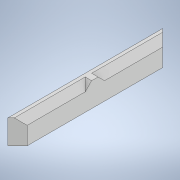
# Autodesk Inventor part: edge-join-no-hole
Saved by Autodesk Inventor 2021 (Build 250183000, 183)
## iProperties
Created: 2020-12-10
Part Number: edge-join-no-hole
Material: Generic
Document SubType Name: Modeling
Designer: Luke Kamols
Density: 1 g/cm^3
Appearance: Default
Author: Luke Kamols
Autodesk Inventor part; units mm, degrees
ref_plane "YZ Plane" through (0, 0, 0) normal (1, 0, 0) x (0, 1, 0)
ref_plane "XZ Plane" through (0, 0, 0) normal (0, 1, 0) x (-1, 0, 0)
ref_plane "XY Plane" through (0, 0, 0) normal (0, 0, 1) x (1, 0, 0)
sketch "Sketch1" plane through (0, 0, 0) normal (0, 0, 1) x (1, 0, 0)
  line L0 (0, 0) -> (6, 0)
  line L1 (6, 0) -> (6, 11)
  line L2 (0, 0) -> (0, 15)
  line L3 (0, 15) -> (2, 15)
  line L4 (2, 15) -> (6, 11)
  dimension "d0" = 6
  dimension "d1" = 11
  dimension "d2" = 15
  dimension "d3" = 2
  constraints: 10 end point, 2 perpendicular, 1 horizontal, 1 vertical
  measures "d0" distance of L0.start L0.end
  measures "d1" distance of L0.end L1.end
  measures "d2" distance of L0.start L2.end
  measures "d3" distance of L2.end L3.end
extrude "Extrusion1" add sketch "Sketch1" along normal blind 96
sketch "Sketch2" plane through (0, 0, 0) normal (0, -1, 0) x (1, 0, 0)
  line L0 (0, 0) -> (0, 96) projected
  line L1 (5.9866, 0) -> (0, 0)
  line L2 (0, 96) -> (6, 96) projected
  line L3 (0, 96) -> (6, 96)
  line L4 (6, 96) -> (6, 90)
  line L5 (6, 90) -> (0, 96)
  line L6 (0, 0) -> (6, 0) projected
  line L7 (6, 0) -> (0, 0)
  line L8 (6, 0) -> (6, 6)
  line L9 (6, 0) -> (6, 96) projected
  line L10 (6, 6) -> (0, 0)
  dimension "d7" = 6
  dimension "d8" = 6
  constraints: 14 end point, 2 horizontal, 1 collinear, 1 point on line
  measures "d7" distance of L2.end L4.end
  measures "d8" distance of L6.end L8.end
extrude "Extrusion2" cut sketch "Sketch2" against normal blind 42.1125 contours L10 L8 L6 L1 | L2 L4 L5
sketch "Sketch3" plane through (6, 0, 90) normal (1, 0, 0) x (0, 0, -1)
  line L0 (84, 11) -> (0, 11) projected
  line L1 (84, 0) -> (0, 0) projected
  line L2 (42, 11) -> (42, 0)
  line L3 (42, 0) -> (48, 0)
  line L4 (90, 0) -> (-6, 0) projected
  line L5 (48, 0) -> (48, 11)
  line L6 (42, 0) -> (36, 0)
  line L7 (36, 0) -> (36, 11)
  line L8 (42, 11) -> (42, 15)
  line L9 (88, 15) -> (-4, 15) projected
  line L10 (42, 15) -> (44, 15)
  line L11 (44, 15) -> (48, 11)
  line L12 (42, 15) -> (40, 15)
  line L13 (40, 15) -> (36, 11)
  point P0 (36, 0)
  dimension "d11" = 6
  dimension "d12" = 6
  dimension "d13" = 2
  dimension "d14" = 2
  constraints: 20 end point, 5 point on line, 3 midpoint, 3 perpendicular
  measures "d11" distance of L2.end L3.end
  measures "d12" distance of L2.end L6.end
  measures "d13" distance of L8.end L10.end
  measures "d14" distance of L8.end L12.end
extrude "Extrusion3" add sketch "Sketch3" against normal blind 6
body "Solid1"
